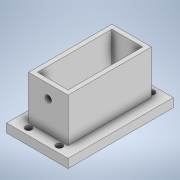
# Autodesk Inventor part: Lens Holder
Saved by Autodesk Inventor 2022 (Build 260153000, 153)
## iProperties
Created: 2023-09-18
Part Number: Lens Holder
Material: Generic
Document SubType Name: Modeling
Designer: fouad
Density: 1 g/cm^3
Appearance: Default
Author: fouad
Autodesk Inventor part; units mm, degrees
ref_plane "YZ Plane" through (0, 0, 0) normal (1, 0, 0) x (0, 1, 0)
ref_plane "XZ Plane" through (0, 0, 0) normal (0, 1, 0) x (-1, 0, 0)
ref_plane "XY Plane" through (0, 0, 0) normal (0, 0, 1) x (1, 0, 0)
sketch "Sketch1" plane through (0, 0, 0) normal (0, 1, 0) x (-1, 0, 0)
  line L0 (6.8865, 9.2769) -> (-0.1135, 9.2769)
  line L1 (-0.1135, 9.2769) -> (-0.1135, -2.7231)
  line L2 (-0.1135, -2.7231) -> (6.8865, -2.7231)
  line L3 (6.8865, -2.7231) -> (6.8865, 9.2769)
  line L4 (5.1365, 7.5269) -> (1.6365, 7.5269)
  line L5 (1.6365, 7.5269) -> (1.6365, -0.9731)
  line L6 (1.6365, -0.9731) -> (5.1365, -0.9731)
  line L7 (5.1365, -0.9731) -> (5.1365, 7.5269)
  point P0 (0, 0)
  dimension "d0" = 7
  dimension "d1" = 12
  dimension "d2" = 1.75
  constraints: 16 end point, 4 parallel, 2 perpendicular, 1 horizontal, 3 other
  measures "d0" distance of L2.end L1.end
  measures "d1" distance of L1.end L0.end
  measures "d2" distance between parallel lines of L3 L7
extrude "Extrusion1" add sketch "Sketch1" along normal blind 1
sketch "Sketch2" plane through (0, 1, 0) normal (0, 1, 0) x (1, 0, 0)
  line L0 (-5.1365, -7.5269) -> (-5.1365, 0.9731) projected
  line L1 (-1.6365, -7.5269) -> (-5.1365, -7.5269) projected
  line L2 (-1.6365, 0.9731) -> (-1.6365, -7.5269) projected
  line L3 (-5.1365, 0.9731) -> (-1.6365, 0.9731) projected
  line L4 (-5.6365, 1.4731) -> (-5.6365, -8.0269)
  line L5 (-5.6365, -8.0269) -> (-1.1365, -8.0269)
  line L6 (-1.1365, -8.0269) -> (-1.1365, 1.4731)
  line L7 (-1.1365, 1.4731) -> (-5.6365, 1.4731)
  line L8 (-5.1365, -7.5269) -> (-1.6365, -7.5269)
  line L9 (-1.6365, -7.5269) -> (-1.6365, 0.9731)
  line L10 (-1.6365, 0.9731) -> (-5.1365, 0.9731)
  line L11 (-5.1365, 0.9731) -> (-5.1365, -7.5269)
  point P0 (0, 0)
  dimension "d5" = 0.5
  constraints: 16 end point, 2 parallel, 1 horizontal, 1 perpendicular, 3 other
  measures "d5" distance between parallel lines of L0 L4
extrude "Extrusion2" add sketch "Sketch2" along normal blind 5
sketch "Sketch3" plane through (0, 1, 0) normal (0, 1, 0) x (1, 0, 0)
  circle A0 centre (-5.1365, -8.5269) radius 0.375
  line L0 (-6.8865, -9.2769) -> (0.1135, -9.2769) projected
  line L1 (-6.8865, 2.7231) -> (-6.8865, -9.2769) projected
  circle A1 centre (-1.6365, -8.5269) radius 0.375
  circle A2 centre (-5.1365, 1.9731) radius 0.375
  circle A3 centre (-1.6365, 1.9731) radius 0.375
  point P0 (0, 0)
  dimension "d8" = 0.75
  dimension "d9" = 0.75
  dimension "d10" = 1.75
  dimension "d13" = 3.5
  dimension "d16" = 10.5
  constraints: 4 centre point, 1 horizontal, 1 vertical, 6 other
  measures "d8" diameter of A0
  measures "d9" distance from line of L0 A0.centre
  measures "d10" distance from line of L1 A0.centre
  measures "d13" distance of A0.centre A1.centre
  measures "d16" distance of A0.centre A2.centre
extrude "Extrusion3" cut sketch "Sketch3" against normal blind 5
sketch "Sketch6" plane through (-5.6365, 1, 8.0269) normal (0, 0, 1) x (1, 0, 0)
  circle A0 centre (2.25, 3.5) radius 0.375
  line L0 (0, 5) -> (4.5, 5) projected
  line L1 (4.5, 0) -> (4.5, 5) projected
  point P0 (5.6365, -1)
  dimension "d21" = 0.75
  dimension "d22" = 1.5
  dimension "d24" = 2.25
  constraints: 1 centre point
  measures "d21" diameter of A0
  measures "d22" distance from line of L0 A0.centre
  measures "d24" distance from line of L1 A0.centre
extrude "Extrusion4" cut sketch "Sketch6" against normal blind 0.5
body "Solid1"
